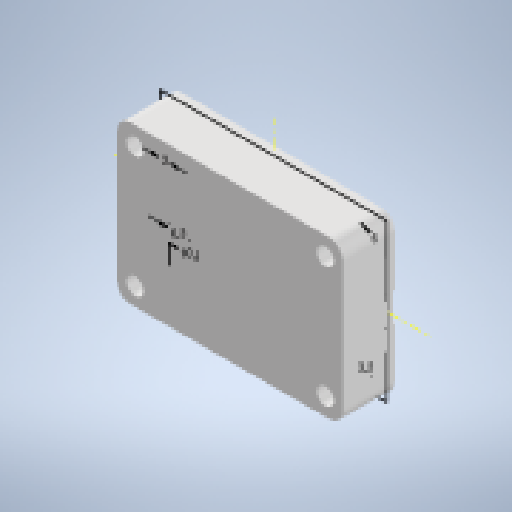
# Autodesk Inventor part: enclosure
Saved by Autodesk Inventor 2025 (Build 290162000, 162)
## iProperties
Created: 2026-02-25
Part Number: enclosure
Material: 一般
Document SubType Name: Modeling
Designer: sooo1
Density: 1 g/cm^3
Appearance: 既定
Author: sooo1
Autodesk Inventor part; units mm, degrees
sketch "スケッチ1" plane through (0, 0, 0) normal (0, 0, 1) x (1, 0, 0)
  line L0 (36, 24) -> (36, -24) construction
  line L1 (-36, 24) -> (36, 24) construction
  line L2 (-36, -24) -> (-36, 24) construction
  line L3 (36, -24) -> (-36, -24) construction
  circle A0 centre (-33, 21) radius 1.5 construction
  circle A1 centre (-33, -21) radius 1.5 construction
  circle A2 centre (33, 21) radius 1.5 construction
  circle A3 centre (33, -21) radius 1.5 construction
  line L4 (-36.3, 24.3) -> (36.3, 24.3)
  line L5 (36.3, 24.3) -> (36.3, -24.3)
  line L6 (36.3, -24.3) -> (-36.3, -24.3)
  line L7 (-36.3, -24.3) -> (-36.3, 24.3)
  circle A4 centre (-33, -21) radius 1.6
  circle A5 centre (-33, 21) radius 1.6
  circle A6 centre (33, -21) radius 1.6
  circle A7 centre (33, 21) radius 1.6
  line L8 (-39.3, 27.3) -> (39.3, 27.3)
  line L9 (39.3, 27.3) -> (39.3, -27.3)
  line L10 (39.3, -27.3) -> (-39.3, -27.3)
  line L11 (-39.3, -27.3) -> (-39.3, 27.3)
  line L12 (-36.3, -14.3) -> (-26.3, -14.3)
  line L13 (-26.3, -14.3) -> (-26.3, -24.3)
  line L14 (-55.02, 0) -> (55.02, 0) construction
  line L15 (0, -38.22) -> (0, 38.22) construction
  line L16 (-36.3, 14.3) -> (-26.3, 14.3)
  line L17 (-26.3, 14.3) -> (-26.3, 24.3)
  line L18 (36.3, -14.3) -> (26.3, -14.3)
  line L19 (26.3, -14.3) -> (26.3, -24.3)
  line L20 (26.3, 14.3) -> (26.3, 24.3)
  line L21 (36.3, 14.3) -> (26.3, 14.3)
  line L22 (22, 5) -> (29, 5) construction
  line L23 (29, -5) -> (22, -5) construction
  line L24 (36, 24) -> (36, -24) projected
  line L25 (36, -24) -> (-36, -24) projected
  line L26 (-36, -24) -> (-36, 24) projected
  line L27 (-36, 24) -> (36, 24) projected
  circle A8 centre (-33, 21) radius 1.5 projected
  circle A9 centre (-33, -21) radius 1.5 projected
  circle A10 centre (33, 21) radius 1.5 projected
  circle A11 centre (33, -21) radius 1.5 projected
  line L28 (39.3, 5) -> (36.3, 5)
  line L29 (39.3, -5) -> (36.3, -5)
  circle A12 centre (33, 21) radius 3
  circle A13 centre (33, -21) radius 3
  circle A14 centre (-33, 21) radius 3
  circle A15 centre (-33, -21) radius 3
  point P0 (0, 0)
  dimension "d0" = 0.3
  dimension "d1" = 3.2
  dimension "d2" = 3
  dimension "d7" = 10
  dimension "d16" = 6
  constraints: 40 end point, 12 symmetric about line, 8 centre point, 6 point on line, 4 perpendicular, 3 equal radius, 3 horizontal, 2 collinear, 13 other
  measures "d0" distance between parallel lines of L2 L7
  measures "d1" diameter of A6
  measures "d2" distance between parallel lines of L7 L11
  measures "d7" distance of L12.start L12.end
  measures "d16" diameter of A12
extrude "押し出し1" add sketch "スケッチ1" along normal blind 7 and the other way blind 3 contours L7 L6 L5 L29 L9 L10 L11 L8 L28 L4 | L28 L9 L29 L5
ref_plane "作業平面1" through (-36, -24, 0) normal (0, 0, 1) x (1, 0, 0)
extrude "押し出し3" add sketch "スケッチ1" against normal up to surface (7 mm away) from surface at 7 contours L4 L17 L27 L26 L16 L7 | L4 L5 L21 L24 L27 L20 | L17 L16 L26 A14 L27 | L12 L26 L25 L13 L6 L7 | L27 A12 L24 L21 L20 | A14 L26 L27 | A14 | L12 L13 L25 A15 L26 | L27 L24 A12 | A12 | A15 L25 L26 | A15 | L19 L25 L24 L18 L5 L6 | L24 A13 L25 L19 L18 | A13 | L24 L25 A13
extrude "押し出し4" add sketch "スケッチ1" along normal blind 3 from surface at 7 contours L7 L6 L5 L29 L9 L10 L11 L8 L28 L4 | L4 L17 L27 L26 L16 L7 | L4 L20 L27 L17 | L16 L26 L12 L7 | L4 L5 L21 L24 L27 L20 | L27 L20 L21 L24 L18 L19 L25 L13 L12 L26 L16 L17 | L17 L16 L26 A14 L27 | L12 L26 L25 L13 L6 L7 | L27 A12 L24 L21 L20 | A14 L26 L27 | A14 | L12 L13 L25 A15 L26 | L5 L18 L24 L21 | L27 L24 A12 | A12 | L13 L25 L19 L6 | A15 L25 L26 | A15 | L28 L9 L29 L5 | L19 L25 L24 L18 L5 L6 | L24 A13 L25 L19 L18 | A13 | L24 L25 A13
ref_plane "作業平面2" through (-39.3, -27.3, -10) normal (0, 0, 1) x (1, 0, 0)
ref_plane "作業平面3" through (-36, -24, -2) normal (0, 0, -1) x (0, 1, 0)
sketch "スケッチ4" plane through (0, 0, 0) normal (0, 0, 1) x (1, 0, 0)
  line L0 (36.3, 24.3) -> (36.3, -24.3) projected
  line L1 (39.3, 27.3) -> (39.3, -27.3) projected
  line L2 (39.3, 5) -> (36.3, 5) projected
  line L3 (39.3, -5) -> (36.3, -5) projected
  point P0 (0, 0)
extrude "押し出し5" cut sketch "スケッチ4" along normal up to surface (8 mm away) from surface at -10
sketch "スケッチ5" plane through (-39.3, -27.3, 10) normal (0, 0, 1) x (1, 0, 0)
  circle A0 centre (6.3, 6.3) radius 3 projected
  circle A1 centre (72.3, 6.3) radius 3 projected
  circle A2 centre (72.3, 48.3) radius 3 projected
  circle A3 centre (6.3, 48.3) radius 3 projected
  line L0 (0, 0) -> (0, 54.6) projected
  line L1 (78.6, 0) -> (0, 0) projected
  line L2 (78.6, 54.6) -> (78.6, 0) projected
  line L3 (0, 54.6) -> (78.6, 54.6) projected
  circle A4 centre (72.3, 6.3) radius 1.6 projected
  circle A5 centre (6.3, 6.3) radius 1.6 projected
  circle A6 centre (6.3, 48.3) radius 1.6 projected
  circle A7 centre (72.3, 48.3) radius 1.6 projected
  point P0 (39.3, 27.3)
extrude "押し出し6" add sketch "スケッチ5" along normal blind 5 contours L0 L3 L2 L1
fillet "フィレット1" radius 5 4 edges at (-39.3, 27.3, 6) (-39.3, -27.3, 6) (39.3, 27.3, 6) (39.3, -27.3, 6)
